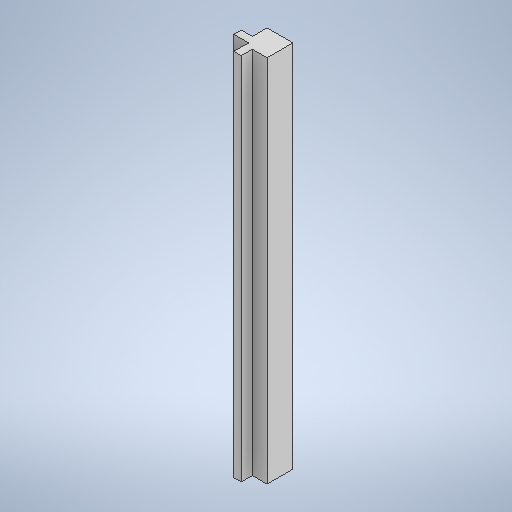
# Autodesk Inventor part: Aluprofil_20x20_H100
Saved by Autodesk Inventor 2025 (Build 290162000, 162)
## iProperties
Created: 2026-06-23
Part Number: Aluprofil_20x20_H100
Material: Generisch
Document SubType Name: Modeling
Designer: GemmiDad-GBSE
Density: 1 g/cm^3
Appearance: Vorgabe
Author: GemmiDad-GBSE
Autodesk Inventor part; units mm, degrees
ref_plane "YZ Plane" through (0, 0, 0) normal (1, 0, 0) x (0, 1, 0)
ref_plane "XZ Plane" through (0, 0, 0) normal (0, 1, 0) x (-1, 0, 0)
sketch "Skizze1" plane through (0, 0, 0) normal (0, 0, 1) x (1, 0, 0)
  line L0 (0, 0) -> (10, 0)
  line L1 (10, 0) -> (10, 10)
  line L2 (10, 10) -> (0, 10)
  line L3 (0, 10) -> (0, 0)
  constraints: 8 end point, 2 parallel, 1 horizontal, 1 perpendicular
extrude "Extrusion1" add sketch "Skizze1" along normal blind 100
sketch "Skizze2" plane through (0, 0, 0) normal (0, 0, 1) x (1, 0, 0)
  line L0 (0, 0) -> (4, 0)
  line L1 (4, 0) -> (4, 4)
  line L2 (4, 4) -> (0, 4)
  line L3 (0, 4) -> (0, 0)
  constraints: 8 end point, 2 parallel, 1 horizontal, 1 perpendicular
extrude "Extrusion2" cut sketch "Skizze2" along normal blind 100
sketch "Skizze3" plane through (0, 0, 0) normal (0, 0, 1) x (1, 0, 0)
  line L0 (-3, 6) -> (3, 6)
  line L1 (3, 6) -> (3, 10)
  line L2 (3, 10) -> (-3, 10)
  line L3 (-3, 10) -> (-3, 6)
  constraints: 8 end point, 2 parallel, 1 horizontal, 1 perpendicular
extrude "Extrusion3" cut sketch "Skizze3" along normal blind 100
sketch "Skizze4" plane through (0, 0, 0) normal (0, 0, 1) x (1, 0, 0)
  line L0 (-3, -10) -> (3, -10)
  line L1 (3, -10) -> (3, -6)
  line L2 (3, -6) -> (-3, -6)
  line L3 (-3, -6) -> (-3, -10)
  constraints: 8 end point, 2 parallel, 1 horizontal, 1 perpendicular
extrude "Extrusion4" cut sketch "Skizze4" along normal blind 100
sketch "Skizze5" plane through (0, 0, 0) normal (0, 0, 1) x (1, 0, 0)
  line L0 (-10, -3) -> (-6, -3)
  line L1 (-6, -3) -> (-6, 3)
  line L2 (-6, 3) -> (-10, 3)
  line L3 (-10, 3) -> (-10, -3)
  constraints: 8 end point, 2 parallel, 1 horizontal, 1 perpendicular
extrude "Extrusion5" cut sketch "Skizze5" along normal blind 100
sketch "Skizze6" plane through (0, 0, 0) normal (0, 0, 1) x (1, 0, 0)
  line L0 (6, -3) -> (10, -3)
  line L1 (10, -3) -> (10, 3)
  line L2 (10, 3) -> (6, 3)
  line L3 (6, 3) -> (6, -3)
  constraints: 8 end point, 2 parallel, 1 horizontal, 1 perpendicular
extrude "Extrusion6" cut sketch "Skizze6" along normal blind 100
ref_plane "Arbeitsebene1" through (0, 0, 100) normal (0, 0, 1) x (1, 0, 0)
sketch "Skizze7" plane through (0, 0, 0) normal (0, 0, 1) x (1, 0, 0)
  circle A0 centre (0, 0) radius 2.5
  constraints: 1 centre point
extrude "Extrusion7" cut sketch "Skizze7" along normal blind 10
sketch "Skizze8" plane through (0, 0, 100) normal (0, 0, 1) x (1, 0, 0)
  circle A0 centre (0, 0) radius 2.5
  constraints: 1 centre point
extrude "Extrusion8" cut sketch "Skizze8" along normal blind 10
